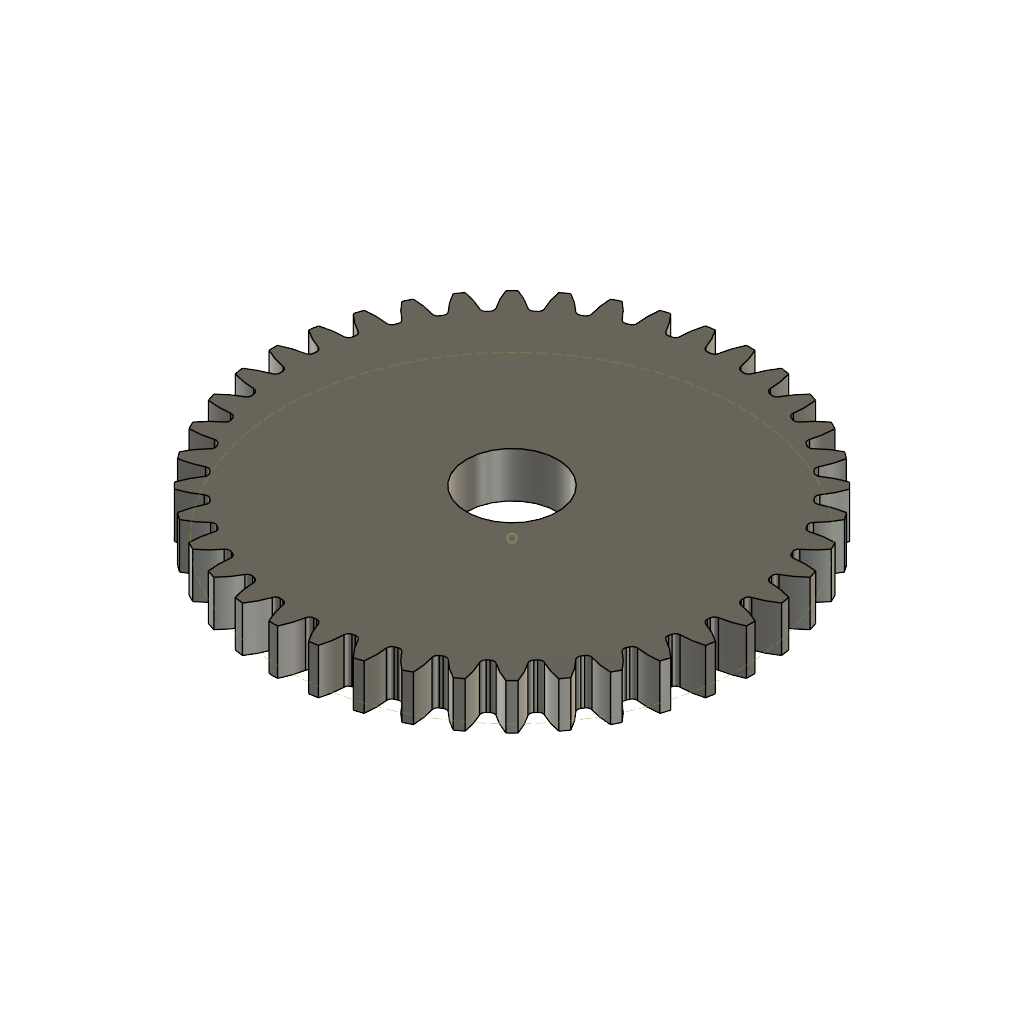
motor gear (Autodesk Fusion 360 design; units mm, degrees)
description: Spur Gear; Module: 0.5; Num Teeth: 40; Pressure Angle: 20.0; Backlash: 0.00 mm
part number: 2026-09-19-16-03-38-792
Autodesk Fusion 360 part; units mm, degrees
sketch "Base Circle" plane through (0, 0, 0) normal (0, 0, 1) x (1, 0, 0)
  circle A0 centre (0, 0) radius 9.4215
  circle A1 centre (0, 0) radius 2
extrude "Extrude1" add sketch "Base Circle" along normal blind 2
sketch "Gear Tooth" plane through (0, 0, 0) normal (0, 0, 1) x (1, 0, 0)
  spline S0 degree 5 poles (9.3831, -0.5088) (9.3863, -0.5089) (9.3927, -0.5089) (9.4023, -0.5088) (9.415, -0.5086) (9.431, -0.5081) (9.4469, -0.5073) (9.4629, -0.5063) (9.4789, -0.505) (9.4949, -0.5035) (9.5109, -0.5018) (9.5269, -0.4999) (9.5428, -0.4978) (9.5588, -0.4956) (9.5749, -0.4933) (9.5909, -0.4909) (9.6069, -0.4883) (9.6229, -0.4856) (9.6389, -0.4827) (9.6549, -0.4797) (9.6709, -0.4766) (9.6869, -0.4734) (9.7029, -0.4701) (9.7189, -0.4667) (9.7349, -0.4631) (9.7509, -0.4595) (9.7669, -0.4557) (9.7829, -0.4519) (9.7989, -0.4479) (9.8149, -0.4439) (9.8309, -0.4397) (9.8469, -0.4355) (9.8629, -0.4311) (9.8788, -0.4267) (9.8948, -0.4222) (9.9108, -0.4176) (9.9268, -0.4129) (9.9428, -0.4081) (9.9587, -0.4032) (9.9747, -0.3982) (9.9906, -0.3931) (10.0066, -0.388) (10.0225, -0.3828) (10.0385, -0.3775) (10.0544, -0.3721) (10.0704, -0.3666) (10.0863, -0.3611) (10.1022, -0.3554) (10.1181, -0.3497) (10.1341, -0.3439) (10.15, -0.338) (10.1659, -0.3321) (10.1818, -0.3261) (10.1977, -0.32) (10.2136, -0.3138) (10.2294, -0.3075) (10.2453, -0.3012) (10.2612, -0.2948) (10.277, -0.2883) (10.2929, -0.2818) (10.3087, -0.2752) (10.3246, -0.2685) (10.3404, -0.2617) (10.3562, -0.2549) (10.372, -0.248) (10.3878, -0.241) (10.4036, -0.2339) (10.4194, -0.2268) (10.4352, -0.2196) (10.451, -0.2124) (10.4668, -0.205) (10.4794, -0.1991) (10.4888, -0.1946) (10.4951, -0.1917) (10.4983, -0.1902) knots 0 0 0 0 0 0 0.01428571 0.02857143 0.04285714 0.05714286 0.07142857 0.08571429 0.1 0.11428571 0.12857143 0.14285714 0.15714286 0.17142857 0.18571429 0.2 0.21428571 0.22857143 0.24285714 0.25714286 0.27142857 0.28571429 0.3 0.31428571 0.32857143 0.34285714 0.35714286 0.37142857 0.38571429 0.4 0.41428571 0.42857143 0.44285714 0.45714286 0.47142857 0.48571429 0.5 0.51428571 0.52857143 0.54285714 0.55714286 0.57142857 0.58571429 0.6 0.61428571 0.62857143 0.64285714 0.65714286 0.67142857 0.68571429 0.7 0.71428571 0.72857143 0.74285714 0.75714286 0.77142857 0.78571429 0.8 0.81428571 0.82857143 0.84285714 0.85714286 0.87142857 0.88571429 0.9 0.91428571 0.92857143 0.94285714 0.95714286 0.97142857 0.98571429 1 1 1 1 1 1
  spline S1 degree 5 poles (9.3831, 0.5088) (9.3863, 0.5089) (9.3927, 0.5089) (9.4023, 0.5088) (9.415, 0.5086) (9.431, 0.5081) (9.4469, 0.5073) (9.4629, 0.5063) (9.4789, 0.505) (9.4949, 0.5035) (9.5109, 0.5018) (9.5269, 0.4999) (9.5428, 0.4978) (9.5588, 0.4956) (9.5749, 0.4933) (9.5909, 0.4909) (9.6069, 0.4883) (9.6229, 0.4856) (9.6389, 0.4827) (9.6549, 0.4797) (9.6709, 0.4766) (9.6869, 0.4734) (9.7029, 0.4701) (9.7189, 0.4667) (9.7349, 0.4631) (9.7509, 0.4595) (9.7669, 0.4557) (9.7829, 0.4519) (9.7989, 0.4479) (9.8149, 0.4439) (9.8309, 0.4397) (9.8469, 0.4355) (9.8629, 0.4311) (9.8788, 0.4267) (9.8948, 0.4222) (9.9108, 0.4176) (9.9268, 0.4129) (9.9428, 0.4081) (9.9587, 0.4032) (9.9747, 0.3982) (9.9906, 0.3931) (10.0066, 0.388) (10.0225, 0.3828) (10.0385, 0.3775) (10.0544, 0.3721) (10.0704, 0.3666) (10.0863, 0.3611) (10.1022, 0.3554) (10.1181, 0.3497) (10.1341, 0.3439) (10.15, 0.338) (10.1659, 0.3321) (10.1818, 0.3261) (10.1977, 0.32) (10.2136, 0.3138) (10.2294, 0.3075) (10.2453, 0.3012) (10.2612, 0.2948) (10.277, 0.2883) (10.2929, 0.2818) (10.3087, 0.2752) (10.3246, 0.2685) (10.3404, 0.2617) (10.3562, 0.2549) (10.372, 0.248) (10.3878, 0.241) (10.4036, 0.2339) (10.4194, 0.2268) (10.4352, 0.2196) (10.451, 0.2124) (10.4668, 0.205) (10.4794, 0.1991) (10.4888, 0.1946) (10.4951, 0.1917) (10.4983, 0.1902) knots 0 0 0 0 0 0 0.01428571 0.02857143 0.04285714 0.05714286 0.07142857 0.08571429 0.1 0.11428571 0.12857143 0.14285714 0.15714286 0.17142857 0.18571429 0.2 0.21428571 0.22857143 0.24285714 0.25714286 0.27142857 0.28571429 0.3 0.31428571 0.32857143 0.34285714 0.35714286 0.37142857 0.38571429 0.4 0.41428571 0.42857143 0.44285714 0.45714286 0.47142857 0.48571429 0.5 0.51428571 0.52857143 0.54285714 0.55714286 0.57142857 0.58571429 0.6 0.61428571 0.62857143 0.64285714 0.65714286 0.67142857 0.68571429 0.7 0.71428571 0.72857143 0.74285714 0.75714286 0.77142857 0.78571429 0.8 0.81428571 0.82857143 0.84285714 0.85714286 0.87142857 0.88571429 0.9 0.91428571 0.92857143 0.94285714 0.95714286 0.97142857 0.98571429 1 1 1 1 1 1
  arc A0 (10.4983, -0.1902) -> (10.4983, 0.1902) centre (0, 0) ccw
  line L0 (9.3831, 0.5088) -> (9.3831, -0.5088)
  point P0 (9.4622, -0.5063)
  point P1 (9.5415, -0.498)
  point P2 (9.621, -0.4858)
  point P3 (9.7007, -0.4705)
  point P4 (9.7804, -0.4525)
  point P5 (9.8602, -0.4318)
  point P6 (9.9401, -0.4089)
  point P7 (10.0199, -0.3836)
  point P8 (10.0998, -0.3563)
  point P9 (10.1796, -0.3269)
  point P10 (10.2594, -0.2955)
  point P11 (10.3391, -0.2622)
  point P12 (10.4187, -0.2271)
  point P13 (9.4622, 0.5063)
  point P14 (9.5415, 0.498)
  point P15 (9.621, 0.4858)
  point P16 (9.7007, 0.4705)
  point P17 (9.7804, 0.4525)
  point P18 (9.8602, 0.4318)
  point P19 (9.9401, 0.4089)
  point P20 (10.0199, 0.3836)
  point P21 (10.0998, 0.3563)
  point P22 (10.1796, 0.3269)
  point P23 (10.2594, 0.2955)
  point P24 (10.3391, 0.2622)
  point P25 (10.4187, 0.2271)
extrude "Extrude2" add sketch "Gear Tooth" along normal blind 2
fillet "Fillet1" radius 0.2 2 edges at (9.4078, 0.5087, 1) (9.4078, -0.5087, 1)
pattern_circular "C-Pattern1" count 40 over 360 about axis through (0, 0, 0) along (0, 0, 1) of "Extrude2", "Fillet1"
sketch "Diametrial Pitch Circle" plane through (0, 0, 0) normal (0, 0, 1) x (1, 0, 0)
  circle A0 centre (0, 0) radius 10 construction
named bodies: "motor gear"
